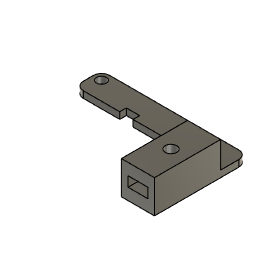
pcb holder (Autodesk Fusion 360 design; units mm, degrees)
Autodesk Fusion 360 part; units mm, degrees
sketch "Sketch1" plane through (0, 0, 0) normal (0, 0, 1) x (1, 0, 0)
  line L0 (0, 0) -> (44, 0)
  line L1 (44, 0) -> (44, -8)
  line L2 (44, -8) -> (0, -8)
  line L3 (0, -8) -> (0, 0)
  line L4 (44, -8) -> (34, -8)
  line L5 (34, -8) -> (34, -28)
  line L6 (34, -28) -> (44, -28)
  line L7 (44, -28) -> (44, -8)
  circle A0 centre (2.5, -2.5) radius 1.5
  line L8 (2.5, -2.5) -> (2.5, 0) construction
  line L9 (2.5, -2.5) -> (0, -2.5) construction
  line L10 (13.5, -8) -> (17.5, -8)
  line L11 (17.5, -8) -> (17.5, -6)
  line L12 (17.5, -6) -> (13.5, -6)
  line L13 (13.5, -6) -> (13.5, -8)
  point P0 (15.5, -6)
  dimension "d1" = 3
  dimension "d2" = 2.5
  dimension "d3" = 8
  dimension "d4" = 13
  dimension "d5" = 2
  dimension "d6" = 4
  dimension "d7" = 44
  dimension "d9" = 20
  dimension "d23" = 34
  constraint horizontal L0
  constraint vertical L1
  constraint horizontal L2
  constraint vertical L3
  constraint coincident L0.start L3.end
  constraint horizontal L4
  constraint vertical L5
  constraint horizontal L6
  constraint vertical L7
  constraint coincident A0.centre L8.start
  constraint coincident L0 L8.end
  constraint perpendicular L0 L8
  constraint coincident L3 L9.end
  constraint perpendicular L3 L9
  constraint equal L8 L9
  constraint horizontal L10
  constraint vertical L11
  constraint horizontal L12
  constraint vertical L13
  constraint coincident L2 L10.start
  constraint midpoint L12 P0
  measures "d1" diameter of A0
  measures "d2" distance of L0 A0.centre
  measures "d3" distance of L0.start L2.end
  measures "d4" horizontal distance of A0.centre P0
  measures "d5" distance of L2 L12
  measures "d6" distance of L11 L13
  measures "d7" distance of L1 L3
  measures "d9" distance of L4 L6
  measures "d23" distance of L3 L5
extrude "Extrude1" add sketch "Sketch1" along normal blind 2 contours L0 L1 L2 L3 L4 L11 L12 L13 | L2 L4 L5 L6 L7
extrude "Extrude2" add sketch "Sketch1" along normal blind 10 contours L2 L4 L5 L6 L7
fillet "Fillet1" radius 2.5 3 edges at (0, 0, 1) (0, -8, 1) (44, 0, 1)
sketch "Sketch2" plane through (0, -28, 0) normal (0, -1, 0) x (1, 0, 0)
  line L0 (34, 0) -> (44, 0)
  line L1 (44, 0) -> (44, 10)
  line L2 (44, 10) -> (34, 10)
  line L3 (34, 10) -> (34, 0)
  line L4 (34, 10) -> (44, 0) construction
  line L5 (36, 3.5) -> (42, 6.5) construction
  line L6 (36, 3.5) -> (42, 3.5)
  line L7 (42, 3.5) -> (42, 6.5)
  line L8 (42, 6.5) -> (36, 6.5)
  line L9 (36, 6.5) -> (36, 3.5)
  dimension "d17" = 6
  dimension "d18" = 3
  constraint coincident L2.end L3.start
  constraint coincident L0.end L1.start
  constraint midpoint L4 L5
  constraint horizontal L6
  constraint vertical L7
  constraint horizontal L8
  constraint vertical L9
  measures "d17" distance of L5.end L8.end
  measures "d18" distance of L5.end L6.end
extrude "Extrude3" cut sketch "Sketch2" against normal through all contours L6 L7 L8 L9
sketch "Sketch3" plane through (0, 0, 10) normal (0, 0, 1) x (-1, 0, 0)
  line L0 (-44, 28) -> (-44, 8)
  line L1 (-44, 8) -> (-34, 8)
  line L2 (-34, 8) -> (-34, 28)
  line L3 (-34, 28) -> (-44, 28)
  line L4 (-34, 8) -> (-44, 28) construction
  circle A0 centre (-39, 18) radius 1.75
  dimension "d20" = 3.5
  constraint coincident L1.end L2.start
  constraint coincident L0.start L3.end
  constraint midpoint L4 A0.centre
  measures "d20" diameter of A0
extrude "Extrude4" cut sketch "Sketch3" against normal up to surface (6.5 mm away) contours A0
